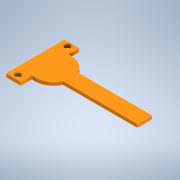
# Autodesk Inventor part: T
Saved by Autodesk Inventor 2021 (Build 250183000, 183)
## iProperties
Created: 2022-11-01
Part Number: T
Material: Generic
Document SubType Name: Modeling
Designer: USUARIO
Density: 1 g/cm^3
Appearance: Orange
Author: USUARIO
Autodesk Inventor part; units mm, degrees
ref_plane "YZ Plane" through (0, 0, 0) normal (1, 0, 0) x (0, 1, 0)
ref_plane "XZ Plane" through (0, 0, 0) normal (0, 1, 0) x (-1, 0, 0)
ref_plane "XY Plane" through (0, 0, 0) normal (0, 0, 1) x (1, 0, 0)
sketch "Sketch1" plane through (0, 0, 0) normal (0, 1, 0) x (-1, 0, 0)
  line L0 (-140, 10) -> (-10, 10)
  line L1 (-10, 10) -> (-10, -10)
  line L2 (-10, -10) -> (-140, -10)
  line L3 (-140, -10) -> (-140, 10)
  line L4 (-140, 10) -> (-10, -10) construction
  line L5 (-10, 10) -> (-140, -10) construction
  line L6 (10, 40) -> (-10, 40)
  line L7 (-10, 40) -> (-10, -40)
  line L8 (-10, -40) -> (10, -40)
  line L9 (10, -40) -> (10, 40)
  line L10 (10, 40) -> (-10, -40) construction
  line L11 (-10, 40) -> (10, -40) construction
  line L12 (40, 0) -> (-170, 0) projected
  line L13 (0, -56) -> (0, 56) projected
  circle A0 centre (-15, 0) radius 25
  circle A1 centre (0, 34) radius 4
  circle A2 centre (0, -34) radius 4
  point P0 (0, 0)
  point P1 (-75, 0)
  point P2 (0, 0)
  point P3 (-75, 0)
  point P4 (0, 0)
  point P5 (0, 0)
  point P6 (-37.9129, -10)
  point P7 (-10, -24.4949)
  point P8 (-10, 24.4949)
  point P9 (-37.9129, 10)
  dimension "d0" = 20
  dimension "d1" = 20
  dimension "d2" = 80
  dimension "d3" = 150
  dimension "d5" = 50
  dimension "d6" = 15
  dimension "d7" = 8
  dimension "d8" = 6
  dimension "d9" = 8
  dimension "d10" = 6
  constraints: 24 end point, 8 midpoint, 6 point on line, 4 parallel, 3 centre point, 2 horizontal, 2 perpendicular
  measures "d0" distance between parallel lines of L7 L9
  measures "d1" distance of L2.end L0.start
  measures "d2" distance of L8.end L6.start
  measures "d3" distance between parallel lines of L3 L9
  measures "d5" diameter of A0
  measures "d6" distance of point (0, 0) A0.centre
  measures "d7" diameter of A1
  measures "d8" distance from line of L6 A1.centre
  measures "d9" diameter of A2
  measures "d10" distance from line of L8 A2.centre
extrude "Extrusion1" add sketch "Sketch1" along normal blind 5 contours L0 A0 L12 L3 | A0 L7 L0 | L0 L1 L12 A0 | L12 A0 L2 L3 | L7 A0 L13 L12 L1 | L7 L6 L13 A1 A0 | L12 L1 L2 A0 | L12 L13 A0 L7 L1 | A0 L12 L13 | L13 A1 L6 L9 A0 | L2 L7 A0 | L12 A0 L13 | L9 L8 L13 A2 A0 | A0 L13 A2 L8 L7
equation "\"d0\" = AnEsl"
equation "\"d1\" = AnEsl"
equation "\"d9\" = d7"
equation "\"d10\" = d8"
equation "\"AnEsl\" = 20"
body "Solid1"
